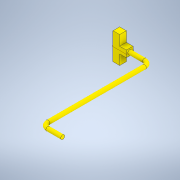
# Autodesk Inventor part: gancho
Saved by Autodesk Inventor 2021.1 (Build 251245000, 245)
## iProperties
Created: 2020-12-31
Part Number: gancho
Material: Generic
Document SubType Name: Modeling
Designer: Bolisteward
Density: 1 g/cm^3
Appearance: Default
Author: Bolisteward
Autodesk Inventor part; units mm, degrees
ref_plane "YZ Plane" through (0, 0, 0) normal (1, 0, 0) x (0, 1, 0)
ref_plane "XY Plane" through (0, 0, 0) normal (0, 0, 1) x (1, 0, 0)
sketch "Sketch1" plane through (0, 0, 0) normal (0, 0, 1) x (1, 0, 0)
  line L0 (0, 0) -> (5, 0)
  line L1 (5, 0) -> (5, 20)
  line L2 (5, 20) -> (0, 20)
  line L3 (0, 20) -> (0, 0)
  line L4 (5, 12.5) -> (10, 12.5)
  line L5 (10, 12.5) -> (10, 7.5)
  line L6 (10, 7.5) -> (5, 7.5)
  line L7 (5, 7.5) -> (5, 12.5)
  line L8 (0, 10) -> (28.6549, 10) construction
  dimension "d0" = 5
  dimension "d1" = 20
  dimension "d2" = 5
  dimension "d3" = 5
  dimension "d4" = 2.5
  constraints: 18 end point, 4 parallel, 3 horizontal, 2 perpendicular, 1 midpoint, 1 point on line
  measures "d0" distance of L2.end L1.end
  measures "d1" distance of L1.end L0.end
  measures "d2" distance of L5.end L6.end
  measures "d3" distance of L4.end L5.end
  measures "d4" distance between parallel lines of L6 L8
extrude "Extrusion1" add sketch "Sketch1" along normal blind 5
ref_plane "Work Plane2" through (0, 10, 0) normal (0, 1, 0) x (-1, 0, 0)
sketch "Sketch2" plane through (0, 10, 0) normal (0, 1, 0) x (-1, 0, 0)
  line L0 (-10, 0) -> (-10, 5) projected
  line L1 (-10, 2.5) -> (-21, 2.5)
  line L2 (-25, 6.5) -> (-25, 78.5)
  line L3 (-29, 82.5) -> (-40, 82.5)
  arc A0 (-25, 6.5) -> (-21, 2.5) centre (-21, 6.5) ccw
  arc A1 (-25, 78.5) -> (-29, 82.5) centre (-29, 78.5) ccw
  point P0 (0, 0)
  dimension "d11" = 8
  dimension "d12" = 8
  dimension "d13" = 15
  dimension "d14" = 80
  dimension "d16" = 15
  constraints: 6 end point, 4 point on circle, 4 tangent, 2 centre point, 2 perpendicular, 1 horizontal, 1 midpoint
  measures "d11" diameter of A0
  measures "d12" diameter of A1
  measures "d13" distance from line of L3.end L2
  measures "d14" distance between parallel lines of L3 L1
  measures "d16" distance between parallel lines of L0 L2
sketch "Sketch3" plane through (10, 7.5, 0) normal (1, 0, 0) x (0, 0, -1)
  circle A0 centre (-2.5, 2.5) radius 1.5
  line L0 (0, 5) -> (-5, 5) projected
  line L1 (0, 0) -> (0, 5) projected
  point P0 (0, -7.5)
  dimension "d17" = 3
  dimension "d18" = 2.5
  dimension "d19" = 2.5
  constraints: 1 centre point
  measures "d17" diameter of A0
  measures "d18" distance from line of A0.centre L0
  measures "d19" distance from line of L1 A0.centre
sweep "Sweep1" add profiles "Sketch3" path "Sketch2" path curves L1 A0 L2 A1 L3
body "Solid1"
